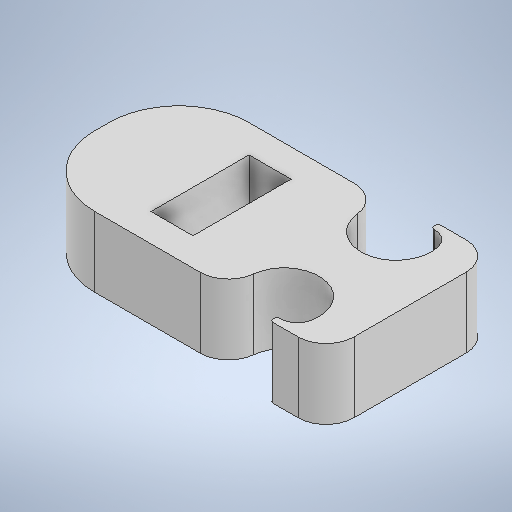
# Autodesk Inventor part: parallel cable holder v2
Saved by Autodesk Inventor 2025.2 (Build 292293000, 293)
## iProperties
Created: 2025-08-07
Part Number: parallel cable holder v2
Material: Generic
Document SubType Name: Modeling
Designer: AkramiLab
Density: 1 g/cm^3
Appearance: Default
Author: AkramiLab
Autodesk Inventor part; units mm, degrees
ref_plane "YZ Plane" through (0, 0, 0) normal (1, 0, 0) x (0, 1, 0)
ref_plane "XZ Plane" through (0, 0, 0) normal (0, 1, 0) x (-1, 0, 0)
ref_plane "XY Plane" through (0, 0, 0) normal (0, 0, 1) x (1, 0, 0)
sketch "Sketch1" plane through (0, 0, 0) normal (0, 1, 0) x (-1, 0, 0)
  line L0 (0, 0) -> (22, 0)
  line L1 (22, 0) -> (22, -11)
  line L2 (22, -11) -> (0, -11)
  line L3 (0, -11) -> (0, 0)
  dimension "d0" = 22
  dimension "d1" = 11
  constraints: 8 end point, 2 parallel, 1 horizontal, 1 perpendicular
  measures "d0" distance of L1.end L2.end
  measures "d1" distance of L0.end L1.end
extrude "Extrusion1" add sketch "Sketch1" along normal blind 5
sketch "Sketch2" plane through (0, 5, 0) normal (0, 1, 0) x (1, 0, 0)
  circle A0 centre (-5, 1.5) radius 2.5
  circle A1 centre (-5, 9.5) radius 2.5
  line L0 (-22, 0) -> (0, 0) projected
  line L1 (0, 11) -> (-22, 11) projected
  line L2 (0, 0) -> (0, 11) projected
  dimension "d4" = 5
  dimension "d5" = 5
  dimension "d6" = 1.5
  dimension "d7" = 1.5
  dimension "d14" = 5
  dimension "d15" = 5
  constraints: 2 centre point
  measures "d4" diameter of A0
  measures "d5" diameter of A1
  measures "d6" distance from line of L0 A0.centre
  measures "d7" distance from line of L1 A1.centre
  measures "d14" distance from line of L2 A0.centre
  measures "d15" distance from line of L2 A1.centre
extrude "Extrusion2" cut sketch "Sketch2" against normal blind 5
fillet "Fillet1" radius 2 1 edges at (-7, 2.5, 0)
fillet "Fillet2" radius 2 1 edges at (-7, 2.5, -11)
fillet "Fillet3" radius 5 1 edges at (-22, 2.5, -11)
fillet "Fillet4" radius 5 1 edges at (-22, 2.5, 0)
sketch "Sketch3" plane through (0, 5, 0) normal (0, 1, 0) x (1, 0, 0)
  line L0 (0, 0) -> (0, 11) projected
  line L1 (0, 11) -> (-4, 11)
  line L2 (-4, 11) -> (-4, 11.5)
  line L3 (-4, 11.5) -> (0, 11.5)
  line L4 (0, 11.5) -> (0, 11)
  line L5 (0, 0) -> (-4, 0)
  line L6 (-4, 0) -> (-4, -0.5)
  line L7 (-4, -0.5) -> (0, -0.5)
  line L8 (0, -0.5) -> (0, 0)
  dimension "d16" = 4
  dimension "d17" = 0.5
  dimension "d18" = 4
  dimension "d19" = 0.5
  constraints: 16 end point, 4 parallel, 2 horizontal, 2 perpendicular
  measures "d16" distance of L2.end L3.end
  measures "d17" distance of L1.end L2.end
  measures "d18" distance of L7.end L6.end
  measures "d19" distance of L6.end L5.end
extrude "Extrusion3" add sketch "Sketch3" against normal blind 5
fillet "Fillet5" radius 1.2 1 edges at (-3, 2.5, 0)
fillet "Fillet6" radius 1.2 1 edges at (-3, 2.5, -11)
fillet "Fillet7" radius 0.2 1 edges at (-4, 2.5, -11)
fillet "Fillet8" radius 0.2 1 edges at (-4, 2.5, -11.5)
fillet "Fillet9" radius 0.2 1 edges at (-4, 2.5, 0)
fillet "Fillet10" radius 0.2 1 edges at (-4, 2.5, 0.5)
fillet "Fillet11" radius 2 1 edges at (0, 2.5, -11.5)
fillet "Fillet12" radius 2 1 edges at (0, 2.5, 0.5)
sketch "Sketch4" plane through (-22, 0, -6) normal (-1, 0, 0) x (0, 0, 1)
  circle A0 centre (0.5, 2.5) radius 1.65
  line L0 (6, 0) -> (6, 5) projected
  line L1 (-5, 5) -> (-5, 0) projected
  point P0 (-5, 2.5)
  dimension "d30" = 3.3
  dimension "d31" = 5.5
  dimension "d33" = 5.5
  constraints: 1 centre point, 1 midpoint
  measures "d30" diameter of A0
  measures "d31" distance from line of A0.centre L0
  measures "d33" distance of A0.centre point (-5, 2.5)
extrude "Extrusion4" cut sketch "Sketch4" against normal blind 5
sketch "Sketch5" plane through (0, 5, 0) normal (0, 1, 0) x (1, 0, 0)
  line L0 (-15, 2) -> (-12, 2)
  line L1 (-12, 2) -> (-12, 9)
  line L2 (-12, 9) -> (-15, 9)
  line L3 (-15, 9) -> (-15, 2)
  line L4 (-17, 0) -> (-9.4721, 0) projected
  line L5 (-9.4721, 11) -> (-17, 11) projected
  line L6 (-22, 6) -> (-22, 5) projected
  point P0 (0, 0)
  point P1 (-13.5, 2)
  point P2 (-13.5, 9)
  point P3 (-22, 5.5)
  point P4 (-15, 5.5)
  dimension "d36" = 2
  dimension "d37" = 2
  dimension "d38" = 7
  dimension "d39" = 3
  constraints: 8 end point, 4 midpoint, 2 parallel, 1 horizontal, 1 perpendicular
  measures "d36" distance from line of L4 point (-13.5, 2)
  measures "d37" distance from line of L5 point (-13.5, 9)
  measures "d38" distance of point (-22, 5.5) point (-15, 5.5)
  measures "d39" distance between parallel lines of L1 L3
extrude "Extrusion5" cut sketch "Sketch5" against normal blind 10
equation "\"d34\" = ScrewDepth"
equation "\"ScrewDepth\" = 5"
body "Solid1"
